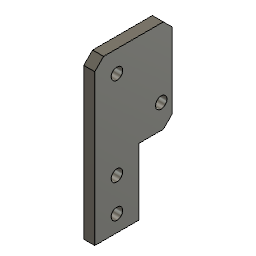
pulley_mount_ed (Autodesk Fusion 360 design; units mm, degrees)
Autodesk Fusion 360 part; units mm, degrees
sketch "Sketch1" plane through (0, 0, 0) normal (1, 0, 0) x (0, 0, -1)
  line L0 (-10, 21) -> (25, 21)
  line L1 (25, 21) -> (25, -21)
  line L2 (25, -21) -> (-10, -21)
  line L3 (-10, -21) -> (-10, 21)
  line L4 (-10, 0) -> (25, 0) construction
  line L5 (0, 20) -> (0, 2.5)
  line L6 (0, 2.5) -> (0, -55) construction
  line L7 (-10, -21) -> (10, -21)
  line L8 (10, -21) -> (10, -51)
  line L9 (10, -51) -> (-10, -51)
  line L10 (-10, -51) -> (-10, -21)
  line L11 (10, -21) -> (10, -20)
  line L12 (10, -20) -> (10, 30) construction
  line L13 (-10, -21) -> (-10, 30) construction
  line L14 (20, -21) -> (20, 32.0321) construction
  line L15 (-20, -21) -> (-20, 30) construction
  circle A0 centre (20, -10) radius 2.6
  circle A1 centre (0, 11.25) radius 2.6
  circle A2 centre (0, -28.5) radius 2.6
  circle A3 centre (0, -43.5) radius 2.6
  dimension "d1" = 35
  dimension "d4" = 42
  dimension "d36" = 20
  dimension "d37" = 30
  dimension "d38" = 10
  dimension "d39" = 10
  dimension "d40" = 5.2
  dimension "d42" = 5.2
  dimension "d43" = 5.2
  dimension "d44" = 5.2
  dimension "d45" = 7.5
  dimension "d46" = 7.5
  constraint horizontal L0
  constraint vertical L1
  constraint vertical L3
  constraint midpoint L3 L4.start
  constraint midpoint L1 L4.end
  constraint coincident L1.end L2.start
  constraint coincident L5.end L6.start
  constraint perpendicular L4 L6
  constraint horizontal L7
  constraint vertical L8
  constraint horizontal L9
  constraint vertical L10
  constraint coincident L2 L3.start
  constraint perpendicular L2 L11
  constraint perpendicular L2 L12
  constraint perpendicular L0 L13
  constraint coincident L2 L14.start
  constraint perpendicular L0 L14
  constraint coincident L2 L15.start
  constraint perpendicular L0 L15
  constraint coincident L14 A0.centre
  constraint midpoint L5 A1.centre
  constraint coincident L6 A2.centre
  constraint coincident L6 A3.centre
  measures "d1" distance of L0.start L0.end
  measures "d4" distance of L0.end L1.end
  measures "d36" distance of L8.end L9.end
  measures "d37" distance of L2.end L9.end
  measures "d38" distance of L13 L15
  measures "d39" distance of L12 L14
  measures "d40" diameter of A0
  measures "d42" diameter of A1
  measures "d43" diameter of A2
  measures "d44" diameter of A3
  measures "d45" vertical distance of L8.end A3.centre
  measures "d46" distance of L2 A2.centre
extrude "Extrude4" add sketch "Sketch1" along normal blind 5
chamfer "Chamfer2" distance 4 angle 45 3 edges at (2.5, 21, -25) (2.5, -21, -25) (2.5, 21, 10)
